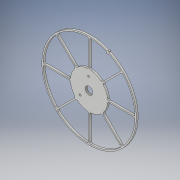
# Autodesk Inventor part: floor
Saved by Autodesk Inventor 2019 (Build 230136000, 136)
## iProperties
Created: 2019-04-16
Part Number: floor
Material: Generic
Document SubType Name: Modeling
Designer: assman
Density: 1 g/cm^3
Appearance: Default
Author: assman
## iProperties of the stored document floor_3DPrint.ipt
Created: 2019-04-16
Part Number: floor_3DPrint
Material: Generic
Document SubType Name: Modeling
Designer: assman
Density: 1 g/cm^3
Appearance: Default
Author: assman
Autodesk Inventor part; units mm, degrees
ref_plane "YZ Plane" through (0, 0, 0) normal (1, 0, 0) x (0, 1, 0)
ref_plane "XZ Plane" through (0, 0, 0) normal (0, 1, 0) x (-1, 0, 0)
ref_plane "XY Plane" through (0, 0, 0) normal (0, 0, 1) x (1, 0, 0)
sketch "Sketch1" plane through (0, 0, 0) normal (0, 0, 1) x (1, 0, 0)
  circle A0 centre (6.7759, 16.1352) radius 1.5 projected
  circle A1 centre (-6.618, -16.2006) radius 1.5 projected
  arc A2 (36.5577, 66.0355) -> (38.9605, 64.9745) centre (7.47, -3.0942) ccw
  line L0 (-5.796, -14.9459) -> (-5.8941, -15.044)
  line L1 (-12.6726, -24.651) -> (-43.4369, -55.4152)
  line L2 (8.47, 69.899) -> (8.47, 26.3918)
  line L3 (6.47, 14.8054) -> (6.47, 14.6667)
  arc A3 (10.9462, 1.7962) -> (8.47, 2.8219) centre (7.47, -3.0942) ccw
  arc A4 (13.3861, -2.0942) -> (12.3604, 0.382) centre (7.47, -3.0942) ccw
  arc A5 (6.47, 2.8219) -> (2.5796, -6.5704) centre (7.47, -3.0942) ccw
  arc A6 (12.3604, -6.5704) -> (13.3861, -4.0942) centre (7.47, -3.0942) ccw
  arc A7 (3.9938, -7.9846) -> (6.47, -9.0102) centre (7.47, -3.0942) ccw
  arc A8 (8.47, -9.0102) -> (10.9462, -7.9846) centre (7.47, -3.0942) ccw
  line L4 (6.47, 17.6037) -> (6.47, 17.465)
  line L5 (-7.7746, -16.9245) -> (-7.8727, -17.0226)
  arc A9 (-12.6726, -24.651) -> (6.47, -32.5801) centre (7.47, -3.0942) ccw
  arc A10 (8.47, -32.5801) -> (27.6126, -24.651) centre (7.47, -3.0942) ccw
  arc A11 (29.0268, -23.2368) -> (36.9559, -4.0942) centre (7.47, -3.0942) ccw
  arc A12 (36.9559, -2.0942) -> (29.0268, 17.0484) centre (7.47, -3.0942) ccw
  arc A13 (27.6126, 18.4626) -> (8.47, 26.3918) centre (7.47, -3.0942) ccw
  arc A14 (6.47, 26.3918) -> (-12.6726, 18.4626) centre (7.47, -3.0942) ccw
  arc A15 (-14.0868, 17.0484) -> (-14.0868, -23.2368) centre (7.47, -3.0942) ccw
  line L6 (19.3867, 23.895) -> (39.0883, 68.5154) construction
  line L7 (19.3867, 23.895) -> (36.9559, 63.6859) construction
  line L8 (35.7859, 64.1904) -> (34.9985, 59.2527)
  line L9 (34.9985, 59.2527) -> (38.1169, 63.1611)
  line L10 (61.2101, 49.2317) -> (61.2054, 49.227)
  line L11 (59.791, 47.8127) -> (29.0268, 17.0484)
  line L12 (59.7959, 50.646) -> (59.7912, 50.6412)
  line L13 (58.3768, 49.2269) -> (27.6126, 18.4626)
  arc A16 (58.3768, 49.2269) -> (38.1169, 63.1611) centre (7.47, -3.0942) ccw
  line L14 (36.9559, -2.0942) -> (80.4631, -2.0942)
  line L15 (82.4633, -2.0942) -> (82.47, -2.0942)
  line L16 (36.9559, -4.0942) -> (80.4631, -4.0942)
  line L17 (82.4633, -4.0942) -> (82.47, -4.0942)
  arc A17 (80.4631, -2.0942) -> (59.791, 47.8127) centre (7.47, -3.0942) ccw
  line L18 (59.7959, -56.8343) -> (59.7912, -56.8296)
  line L19 (58.3768, -55.4152) -> (27.6126, -24.651)
  line L20 (61.2101, -55.4201) -> (61.2054, -55.4154)
  line L21 (59.791, -54.001) -> (29.0268, -23.2368)
  arc A18 (59.791, -54.001) -> (80.4631, -4.0942) centre (7.47, -3.0942) ccw
  line L22 (8.47, -32.5801) -> (8.47, -76.0873)
  line L23 (8.47, -78.0875) -> (8.47, -78.0942)
  line L24 (6.47, -32.5801) -> (6.47, -76.0873)
  line L25 (6.47, -78.0875) -> (6.47, -78.0942)
  arc A19 (8.47, -76.0873) -> (58.3768, -55.4152) centre (7.47, -3.0942) ccw
  line L26 (-14.0868, -23.2368) -> (-44.8511, -54.001)
  line L27 (-46.2654, -55.4154) -> (-46.2701, -55.4201)
  arc A20 (-43.4369, -55.4152) -> (6.47, -76.0873) centre (7.47, -3.0942) ccw
  line L28 (-12.6726, -24.651) -> (-43.4369, -55.4152)
  line L29 (-44.8512, -56.8296) -> (-44.8559, -56.8343)
  line L30 (-67.53, -4.0942) -> (-67.5234, -4.0942)
  line L31 (-65.5232, -4.0942) -> (-22.016, -4.0942)
  line L32 (-67.53, -2.0942) -> (-67.5234, -2.0942)
  line L33 (-65.5232, -2.0942) -> (-22.016, -2.0942)
  arc A21 (-65.5232, -4.0942) -> (-44.8511, -54.001) centre (7.47, -3.0942) ccw
  line L34 (-14.0868, 17.0484) -> (-44.8511, 47.8127)
  line L35 (-46.2654, 49.227) -> (-46.2701, 49.2317)
  line L36 (-12.6726, 18.4626) -> (-43.4369, 49.2269)
  line L37 (-44.8512, 50.6412) -> (-44.8559, 50.646)
  arc A22 (-44.8511, 47.8127) -> (-65.5232, -2.0942) centre (7.47, -3.0942) ccw
  line L38 (6.47, 71.9058) -> (6.47, 71.8992)
  line L39 (6.47, 69.899) -> (6.47, 26.3918)
  arc A23 (35.7859, 64.1904) -> (8.47, 69.899) centre (7.47, -3.0942) ccw
  arc A24 (6.47, 69.899) -> (-43.4369, 49.2269) centre (7.47, -3.0942) ccw
  line L40 (8.47, 71.9058) -> (8.47, 71.8992)
  line L41 (8.47, 69.899) -> (8.47, 26.3918)
  circle A25 centre (7.47, -3.0942) radius 6
  line L42 (36.5577, 66.0355) -> (39.0883, 68.5154)
  line L43 (38.9605, 64.9745) -> (39.0883, 68.5154)
  point P0 (0, 0)
  dimension "d0" = 150
  dimension "d24" = 5
  dimension "d31" = 1.3133
  constraints: 88 end point, 51 point on circle, 23 centre point, 4 coincident, 2 point on line, 1 symmetric about line, 20 other
  measures "d24" distance of L8.start L8.end
  measures "d31" distance from line of L42.start L6
extrude "Extrusion2" add sketch "Sketch1" along normal blind 3
fillet "Fillet1" radius 2 34 edges at (-43.4369, -55.4152, 1.5) (-43.4369, 49.2269, 1.5) (-14.0868, -23.2368, 1.5) (-12.6726, -24.651, 1.5) (6.47, -76.0873, 1.5) (8.47, -76.0873, 1.5) (-65.5232, -4.0942, 1.5) (-65.5232, -2.0942, 1.5) (-22.016, -2.0942, 1.5) (-22.016, -4.0942, 1.5) (6.47, -32.5801, 1.5) (8.47, -32.5801, 1.5) (27.6126, -24.651, 1.5) (29.0268, -23.2368, 1.5) (59.791, -54.001, 1.5) (58.3768, -55.4152, 1.5) (80.4631, -4.0942, 1.5) (80.4631, -2.0942, 1.5) (36.9559, -4.0942, 1.5) (36.9559, -2.0942, 1.5) (29.0268, 17.0484, 1.5) (27.6126, 18.4626, 1.5) (8.47, 26.3918, 1.5) (58.3768, 49.2269, 1.5) (59.791, 47.8127, 1.5) (35.7859, 64.1904, 1.5) (38.1169, 63.1611, 1.5) (8.47, 69.899, 1.5) (6.47, 69.899, 1.5) (-12.6726, 18.4626, 1.5) (-14.0868, 17.0484, 1.5) (-44.8511, 47.8127, 1.5) (-44.8511, -54.001, 1.5) (6.47, 26.3918, 1.5)
fillet "Fillet2" radius 1 1 edges at (34.9985, 59.2527, 1.5)
fillet "Fillet3" radius 1 1 edges at (39.0883, 68.5154, 1.5)
body "Solid2"
